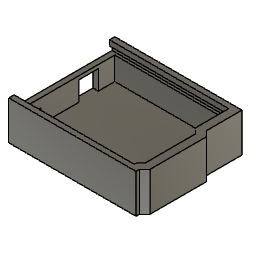
arduino v5 (Autodesk Fusion 360 design; units mm, degrees)
Autodesk Fusion 360 part; units mm, degrees
sketch "Esquisse1" plane through (0, 0, 0) normal (0, 0, 1) x (1, 0, 0) in component "Arduino"
  line L0 (31.2674, 29.4385) -> (-40.7326, 29.4385)
  line L1 (-40.7326, 29.4385) -> (-40.7326, -30.5615)
  line L2 (-40.7326, -30.5615) -> (31.2674, -30.5615)
  line L3 (31.2674, -30.5615) -> (31.2674, -28.5615)
  line L4 (31.2674, -28.5615) -> (34.2674, -25.5615)
  line L5 (34.2674, -25.5615) -> (34.2674, 6.4385)
  line L6 (34.2674, 6.4385) -> (31.2674, 9.4385)
  line L7 (31.2674, 9.4385) -> (31.2674, 29.4385)
  dimension "d8" = 72
  dimension "d9" = 60
  dimension "d10" = 72
  dimension "d11" = 2
  dimension "d12" = 32
  dimension "d14" = 45
  dimension "d15" = 45
  dimension "d16" = 3
  constraint horizontal L0
  constraint perpendicular L0 L1
  constraint perpendicular L1 L2
  constraint perpendicular L2 L3
  constraint perpendicular L0 L7
  measures "d8" distance of L0.start L0.end
  measures "d9" distance of L0.end L1.end
  measures "d10" distance of L1.end L2.end
  measures "d11" distance of L2.end L3.end
  measures "d12" distance of L4.end L5.end
  measures "d14" angle of L2 L4
  measures "d15" angle of L0 L6
  measures "d16" distance of L3 L5
extrude "Extrusion1" add sketch "Esquisse1" along normal blind 13 thin wall 3 inside in component "Arduino"
extrude "Extrusion2" add sketch "Esquisse1" against normal blind 3 in component "Arduino"
sketch "Esquisse1 (2)" plane through (-40.7326, 0, 0) normal (-1, 0, 0) x (0, -1, 0)
  line L0 (30.5615, -3) -> (30.5615, 13)
  line L1 (30.5615, 13) -> (-29.4385, 13)
  line L2 (-29.4385, 13) -> (-29.4385, -3)
  line L3 (-29.4385, -3) -> (30.5615, -3)
  line L4 (-17.1385, 13) -> (-6.1385, 13)
  line L5 (-6.1385, 13) -> (-6.1385, 0)
  line L6 (-6.1385, 0) -> (-17.1385, 0)
  line L7 (-17.1385, 0) -> (-17.1385, 13)
  line L8 (15.3815, 13) -> (24.3815, 13)
  line L9 (24.3815, 13) -> (24.3815, 0)
  line L10 (24.3815, 0) -> (15.3815, 0)
  line L11 (15.3815, 0) -> (15.3815, 13)
  dimension "d26" = 12.3
  dimension "d27" = 3
  dimension "d28" = 11
  dimension "d29" = 13
  dimension "d30" = 3
  dimension "d31" = 6.18
  dimension "d32" = 13
  dimension "d33" = 9
  constraint horizontal L4
  constraint vertical L5
  constraint horizontal L6
  constraint vertical L7
  constraint horizontal L8
  constraint vertical L9
  constraint horizontal L10
  constraint vertical L11
  measures "d26" distance of L2 L7
  measures "d27" distance of L3 L6
  measures "d28" distance of L4.start L4.end
  measures "d29" distance of L4 L6
  measures "d30" distance of L3 L10
  measures "d31" distance of L0 L9
  measures "d32" distance of L8 L10
  measures "d33" distance of L8.start L8.end
extrude "Extrusion3" cut sketch "Esquisse1 (2)" against normal blind 10 contours L1 L8 L9 L10 L11 | L1 L4 L5 L6 L7 in component "Arduino"
sketch "Esquisse2" plane through (0, 0, 13) normal (0, 0, 1) x (-1, 0, 0)
  line L0 (40.7326, -17.1385) -> (37.7326, -17.1385)
  line L1 (37.7326, -17.1385) -> (37.7326, -26.4385)
  line L2 (37.7326, -26.4385) -> (-28.2674, -26.4385)
  line L3 (-28.2674, -26.4385) -> (-28.2674, -8.1959)
  line L4 (-28.2674, -8.1959) -> (-31.2674, -5.1959)
  line L5 (-31.2674, -5.1959) -> (-31.2674, 24.3188)
  line L6 (-31.2674, 24.3188) -> (-28.2674, 27.3188)
  line L7 (-28.2674, 27.3188) -> (-28.2674, 27.5615)
  line L8 (-28.2674, 27.5615) -> (37.7326, 27.5615)
  line L9 (37.7326, 27.5615) -> (37.7326, 24.3815)
  line L10 (37.7326, 24.3815) -> (40.7326, 24.3815)
  line L11 (40.7326, 24.3815) -> (40.7326, 30.5615)
  line L12 (40.7326, 30.5615) -> (-31.2674, 30.5615)
  line L13 (-31.2674, 30.5615) -> (-31.2674, 28.5615)
  line L14 (-31.2674, 28.5615) -> (-34.2674, 25.5615)
  line L15 (-34.2674, 25.5615) -> (-34.2674, -6.4385)
  line L16 (-34.2674, -6.4385) -> (-31.2674, -9.4385)
  line L17 (-31.2674, -9.4385) -> (-31.2674, -29.4385)
  line L18 (-31.2674, -29.4385) -> (40.7326, -29.4385)
  line L19 (40.7326, -29.4385) -> (40.7326, -17.1385)
  line L20 (-31.2674, -29.4385) -> (40.7326, -29.4385)
  line L21 (40.7326, -29.4385) -> (40.7326, -27.9385)
  line L22 (40.7326, -27.9385) -> (-31.2674, -27.9385)
  line L23 (-31.2674, -27.9385) -> (-31.2674, -29.4385)
  line L24 (-31.2674, 30.5615) -> (40.7326, 30.5615)
  line L25 (40.7326, 30.5615) -> (40.7326, 29.0615)
  line L26 (40.7326, 29.0615) -> (-31.2674, 29.0615)
  line L27 (-31.2674, 29.0615) -> (-31.2674, 30.5615)
  dimension "d37" = 1.5
  dimension "d38" = 1.5
  constraint horizontal L20
  constraint vertical L21
  constraint horizontal L22
  constraint vertical L23
  constraint coincident L19 L21.end
  constraint coincident L17.end L18.start
  constraint horizontal L24
  constraint vertical L25
  constraint horizontal L26
  constraint vertical L27
  constraint coincident L11 L25.end
  constraint coincident L12.end L13.start
  measures "d37" distance of L20 L22
  measures "d38" distance of L24 L26
extrude "Extrusion4" add sketch "Esquisse2" along normal blind 6 contours L17 L18 L19 L20 L21 L22 L23 | L11 L12 L13 L24 L25 L26 L27 in component "Arduino"
sketch "Esquisse3" plane through (0, 27.9385, 0) normal (0, -1, 0) x (1, 0, 0)
  line L0 (-40.7326, 13) -> (31.2674, 13)
  line L1 (31.2674, 13) -> (31.2674, 19)
  line L2 (31.2674, 19) -> (-40.7326, 19)
  line L3 (-40.7326, 19) -> (-40.7326, 13)
  line L4 (-40.7326, 19) -> (31.2674, 19)
  line L5 (31.2674, 19) -> (31.2674, 16)
  line L6 (31.2674, 16) -> (-40.7326, 16)
  line L7 (-40.7326, 16) -> (-40.7326, 19)
  dimension "d41" = 3
  constraint horizontal L4
  constraint vertical L5
  constraint horizontal L6
  constraint vertical L7
  constraint coincident L1 L5.end
  constraint coincident L2.end L3.start
  measures "d41" distance of L4 L6
extrude "Extrusion5" add sketch "Esquisse3" along normal blind 1.5 contours L1 L2 L3 L4 L5 L6 L7 in component "Arduino"
sketch "Esquisse4" plane through (0, -29.0615, 0) normal (0, 1, 0) x (-1, 0, 0)
  line L0 (-31.2674, 13) -> (40.7326, 13)
  line L1 (40.7326, 13) -> (40.7326, 19)
  line L2 (40.7326, 19) -> (-31.2674, 19)
  line L3 (-31.2674, 19) -> (-31.2674, 13)
  line L4 (-31.2674, 19) -> (40.7326, 19)
  line L5 (40.7326, 19) -> (40.7326, 16)
  line L6 (40.7326, 16) -> (-31.2674, 16)
  line L7 (-31.2674, 16) -> (-31.2674, 19)
  dimension "d44" = 3
  constraint horizontal L4
  constraint vertical L5
  constraint horizontal L6
  constraint vertical L7
  constraint coincident L1 L5.end
  constraint coincident L2.end L3.start
  measures "d44" distance of L4 L6
extrude "Extrusion6" add sketch "Esquisse4" along normal blind 1.5 contours L1 L2 L3 L4 L5 L6 L7 in component "Arduino"
sketch "Esquisse5" plane through (0, 0, 13) normal (0, 0, 1) x (-1, 0, 0)
  line L0 (-31.2674, -27.9385) -> (40.7326, -27.9385)
  line L1 (40.7326, -27.9385) -> (40.7326, -17.1385)
  line L2 (40.7326, -17.1385) -> (37.7326, -17.1385)
  line L3 (37.7326, -17.1385) -> (37.7326, -26.4385)
  line L4 (37.7326, -26.4385) -> (-28.2674, -26.4385)
  line L5 (-28.2674, -26.4385) -> (-28.2674, -8.1959)
  line L6 (-28.2674, -8.1959) -> (-31.2674, -5.1959)
  line L7 (-31.2674, -5.1959) -> (-31.2674, 24.3188)
  line L8 (-31.2674, 24.3188) -> (-28.2674, 27.3188)
  line L9 (-28.2674, 27.3188) -> (-28.2674, 27.5615)
  line L10 (-28.2674, 27.5615) -> (37.7326, 27.5615)
  line L11 (37.7326, 27.5615) -> (37.7326, 24.3815)
  line L12 (37.7326, 24.3815) -> (40.7326, 24.3815)
  line L13 (40.7326, 24.3815) -> (40.7326, 29.0615)
  line L14 (40.7326, 29.0615) -> (-31.2674, 29.0615)
  line L15 (-31.2674, 29.0615) -> (-31.2674, 28.5615)
  line L16 (-31.2674, 28.5615) -> (-34.2674, 25.5615)
  line L17 (-34.2674, 25.5615) -> (-34.2674, -6.4385)
  line L18 (-34.2674, -6.4385) -> (-31.2674, -9.4385)
  line L19 (-31.2674, -9.4385) -> (-31.2674, -27.9385)
  line L20 (-29.7674, 29.0615) -> (-29.7674, 27.9402)
  line L21 (-29.7674, 27.9402) -> (-32.7674, 24.9402)
  line L22 (-32.7674, 24.9402) -> (-32.7674, -5.8172)
  line L23 (-32.7674, -5.8172) -> (-29.7674, -8.8172)
  line L24 (-29.7674, -8.8172) -> (-29.7674, -27.9385)
  dimension "d47" = -1.5
extrude "Extrusion7" add sketch "Esquisse5" along normal blind 6 contours L0 L14 L15 L16 L17 L18 L19 L20 L21 L22 L23 L24 in component "Arduino"
sketch "Esquisse6" plane through (29.7674, 0, 0) normal (-1, 0, 0) x (0, -1, 0)
  line L0 (-26.4385, 19) -> (-26.4385, 16)
  line L1 (-26.4385, 16) -> (-27.9385, 16)
  line L2 (-27.9385, 16) -> (-27.9385, 13)
  line L3 (-27.9385, 13) -> (-8.8172, 13)
  line L4 (-8.8172, 13) -> (-8.8172, 19)
  line L5 (-8.8172, 19) -> (-26.4385, 19)
  line L6 (-26.4385, 16) -> (-8.8172, 16)
  constraint coincident L0.end L1.start
  constraint midpoint L4 L6.end
sketch "Esquisse7" plane through (19.2923, 19.2923, 0) normal (-0.707107, -0.707107, 0) x (0.707107, -0.707107, 0)
  line L0 (14.8141, 13) -> (19.0567, 13)
  line L1 (19.0567, 13) -> (19.0567, 19)
  line L2 (19.0567, 19) -> (14.8141, 19)
  line L3 (14.8141, 19) -> (14.8141, 13)
  line L4 (14.8141, 16) -> (19.0567, 16)
  constraint midpoint L3 L4.start
  constraint midpoint L1 L4.end
sketch "Esquisse8" plane through (32.7674, 0, 0) normal (-1, 0, 0) x (0, -1, 0)
  line L0 (-5.8172, 13) -> (24.9402, 13)
  line L1 (24.9402, 13) -> (24.9402, 19)
  line L2 (24.9402, 19) -> (-5.8172, 19)
  line L3 (-5.8172, 19) -> (-5.8172, 13)
  line L4 (-5.8172, 16) -> (24.9402, 16)
  constraint midpoint L3 L4.start
  constraint midpoint L1 L4.end
sketch "Esquisse9" plane through (28.8538, -28.8538, 0) normal (-0.707107, 0.707107, 0) x (-0.707107, -0.707107, 0)
  line L0 (-1.2921, 16) -> (-1.8276, 16)
  line L1 (-1.8276, 16) -> (-1.8276, 19)
  line L2 (-1.8276, 19) -> (-5.5347, 19)
  line L3 (-5.5347, 19) -> (-5.5347, 13)
  line L4 (-5.5347, 13) -> (-1.2921, 13)
  line L5 (-1.2921, 13) -> (-1.2921, 16)
  line L6 (-5.5347, 16) -> (-1.2921, 16)
  constraint midpoint L3 L6.start
  constraint coincident L0.start L5.end
extrude "Extrusion8" add sketch "Esquisse6" along normal blind 3 contours L0 L4 L5 L6 in component "Arduino"
extrude "Extrusion9" add sketch "Esquisse7" along normal blind 3 contours L1 L2 L3 L4 in component "Arduino"
extrude "Extrusion10" add sketch "Esquisse8" along normal blind 3 contours L1 L2 L3 L4 in component "Arduino"
extrude "Extrusion11" add sketch "Esquisse9" along normal blind 3 contours L1 L2 L3 L6 in component "Arduino"
revolve "Révolution1" add 1 faces at (28.7674, 8.8172, 17) angle 45 about axis through (29.7674, 8.8172, 16) along (0, 0, 1) in component "Arduino"
revolve "Révolution2" add 1 faces at (28.7319, -26.1473, 17) angle 45 about axis through (30.1461, -27.5615, 19) along (0, 0, 1) in component "Arduino"
sketch "Esquisse10" plane through (0, 23.5938, 0) normal (0, -1, 0) x (1, 0, 0)
  line L0 (-32.2265, 0.0727) -> (-32.2265, 13.0727)
  line L1 (-32.2265, 13.0727) -> (-35.2265, 13.0727)
  line L2 (-35.2265, 13.0727) -> (-35.2265, 0.0727)
  line L3 (-35.2265, 0.0727) -> (-32.2265, 0.0727)
  line L4 (-35.2265, 13.0727) -> (-32.2265, 13.0727)
  line L5 (-32.2265, 13.0727) -> (-32.2265, 11.082)
  line L6 (-32.2265, 11.082) -> (-35.2265, 11.082)
  line L7 (-35.2265, 11.082) -> (-35.2265, 13.0727)
  constraint horizontal L4
  constraint vertical L5
  constraint horizontal L6
  constraint vertical L7
  constraint coincident L0 L5.end
  constraint coincident L1.end L2.start
extrude "Extrusion12" add sketch "Esquisse10" along normal blind 11 contours L0 L1 L2 L4 L5 L6 L7 sketch seen with x (1, 0, 0) y (0, 1, 0) z (0, 0, 1) at (-5.506, -6.4553, -0.0727) in component "Arduino"
sketch "Esquisse11" plane through (0, -8.9262, 0) normal (0, -1, 0) x (1, 0, 0)
  line L0 (-32.2265, 0.0727) -> (-32.2265, 13.0727)
  line L1 (-32.2265, 13.0727) -> (-35.2265, 13.0727)
  line L2 (-35.2265, 13.0727) -> (-35.2265, 0.0727)
  line L3 (-35.2265, 0.0727) -> (-32.2265, 0.0727)
  line L4 (-35.2265, 13.0727) -> (-32.2265, 13.0727)
  line L5 (-32.2265, 13.0727) -> (-32.2265, 8.0552)
  line L6 (-32.2265, 8.0552) -> (-35.2265, 8.0552)
  line L7 (-35.2265, 8.0552) -> (-35.2265, 13.0727)
  constraint horizontal L4
  constraint vertical L5
  constraint horizontal L6
  constraint vertical L7
  constraint coincident L0 L5.end
  constraint coincident L1.end L2.start
extrude "Extrusion13" add sketch "Esquisse11" along normal blind 9 contours L0 L1 L2 L4 L5 L6 L7 sketch seen with x (1, 0, 0) y (0, 1, 0) z (0, 0, 1) at (-5.506, -6.4553, -0.0727) in component "Arduino"
component "Arduino" placed x (1, 0, 0) y (0, 1, 0) z (0, 0, 1) at (5.506, 6.4553, 0.0727)
equation "longueur = 66 mm"
equation "largeur = 54 mm"
equation "epaisseur = 3 mm"
equation "av_long = 3 mm"
equation "av_larg = 32 mm"
equation "av_off_long = 3 mm"
equation "av_off_larg = 2 mm"
equation "d8 = longueur + 2 * epaisseur"
equation "d9 = largeur + 2 * epaisseur"
equation "d10 = longueur + 2 * epaisseur"
equation "d11 = av_off_larg"
equation "d12 = av_larg"
equation "av_angle = 45 deg"
equation "d14 = av_angle"
equation "d15 = av_angle"
equation "d16 = av_off_long"
equation "d17 = epaisseur"
equation "hauteur = 13 mm"
equation "d20 = -epaisseur"
equation "usb_off = 9.3 mm"
equation "pow_off = 3.18 mm"
equation "usb_size = 11 mm"
equation "pow_size = 9 mm"
equation "d26 = epaisseur + usb_off"
equation "d27 = epaisseur"
equation "d28 = usb_size"
equation "d29 = hauteur"
equation "d30 = epaisseur"
equation "d31 = epaisseur + pow_off"
equation "d32 = hauteur"
equation "d33 = pow_size"
equation "ep_plexi = 3 mm"
equation "d37 = epaisseur / 2"
equation "d38 = epaisseur / 2"
equation "d39 = epaisseur + ep_plexi"
equation "d41 = epaisseur"
equation "d42 = epaisseur / 2"
equation "d44 = epaisseur"
equation "d45 = epaisseur / 2"
equation "d47 = -epaisseur / 2"
equation "d48 = epaisseur + ep_plexi"
equation "d50 = epaisseur"
equation "d52 = epaisseur"
equation "d54 = epaisseur"
equation "d56 = epaisseur"
equation "d60 = usb_size"
equation "d62 = pow_size"
